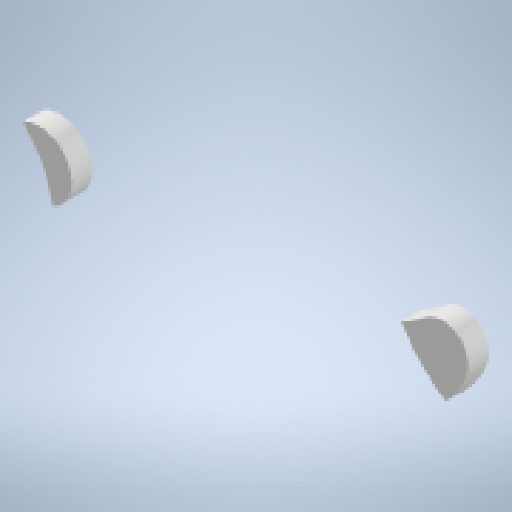
# Autodesk Inventor part: HandsGoma
Saved by Autodesk Inventor 2023 (Build 270158000, 158)
## iProperties
Created: 2022-11-10
Part Number: HandsGoma
Material: Generic
Document SubType Name: Modeling
Designer: reide
Density: 1 g/cm^3
Appearance: Default
Author: reide
Autodesk Inventor part; units mm, degrees
ref_plane "YZ Plane" through (0, 0, 0) normal (1, 0, 0) x (0, 1, 0)
ref_plane "XZ Plane" through (0, 0, 0) normal (0, 1, 0) x (-1, 0, 0)
ref_plane "XY Plane" through (0, 0, 0) normal (0, 0, 1) x (1, 0, 0)
sketch "Sketch1" plane through (0, 0, 0) normal (0, 0, 1) x (1, 0, 0)
  line L0 (0.1525, -4.2135) -> (0.1525, 53.059) projected
  arc A0 (0.5445, -3.1745) -> (-2.4955, 2.7252) centre (-10.3318, -5.0457) ccw projected
  arc A1 (0.5445, -3.1745) -> (-2.4955, 2.7252) centre (-0.8271, -0.1481) ccw projected
  arc A2 (38.4977, -0.5778) -> (40.5936, 2.6407) centre (30.8639, 6.6849) ccw projected
  arc A3 (40.5936, 2.6407) -> (36.4911, 5.8507) centre (38.1416, 3.7335) ccw projected
  arc A4 (33.9966, 4.1943) -> (36.4911, 5.8507) centre (26.9655, 17.4896) ccw projected
  arc A5 (33.9966, 4.1943) -> (38.4977, -0.5778) centre (46.7107, 11.6776) ccw projected
  arc A6 (0.5445, -2.9826) -> (-2.3435, 2.6221) centre (-9.7879, -4.7603) ccw
  arc A7 (0.5445, -2.9826) -> (-2.3435, 2.6221) centre (-0.7585, -0.1076) ccw
  arc A8 (34.2039, 4.1713) -> (38.4799, -0.3622) centre (46.2822, 11.2804) ccw
  arc A9 (40.471, 2.6953) -> (36.5736, 5.7448) centre (38.1416, 3.7335) ccw
  arc A10 (34.2039, 4.1713) -> (36.5736, 5.7448) centre (27.5243, 16.8018) ccw
  arc A11 (38.4799, -0.3622) -> (40.471, 2.6953) centre (31.2278, 6.5373) ccw
  point P0 (0, 0)
  point P1 (0.5445, 0.6626)
  constraints: 12 point on circle, 6 centre point
extrude "Extrusion1" add sketch "Sketch1" along normal blind 2 contours A6 A7 L0 | L0 A7 A6 | A10 A9 A11 A8
body "Solid1"
